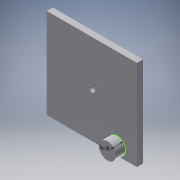
# Autodesk Inventor part: Base
Saved by Autodesk Inventor 2016 SP1 (Build 200210100, 210)
## iProperties
Created: 2016-01-27
Part Number: Base
Material: PVC, non plastifié
Document SubType Name: Modeling
Designer: sd
Density: 1.4 g/cm^3
Appearance: Lisse - Blanc
Author: sd
Autodesk Inventor part; units mm, degrees
ref_plane "YZ Plane" through (0, 0, 0) normal (1, 0, 0) x (0, 1, 0)
ref_plane "XZ Plane" through (0, 0, 0) normal (0, 1, 0) x (-1, 0, 0)
ref_plane "XY Plane" through (0, 0, 0) normal (0, 0, 1) x (1, 0, 0)
sketch "Esquisse1" plane through (0, 0, 0) normal (0, 1, 0) x (-1, 0, 0)
  line L0 (-75, 75) -> (75, 75)
  line L1 (75, 75) -> (75, -75)
  line L2 (75, -75) -> (-75, -75)
  line L3 (-75, -75) -> (-75, 75)
  point P0 (0, 0)
  dimension "d0" = 150
  dimension "d1" = 75
  dimension "d2" = 150
  dimension "d3" = 75
  constraints: 8 end point, 2 parallel, 1 horizontal, 1 perpendicular
  measures "d0" distance of L2.end L0.start
  measures "d1" horizontal distance of point (0, 0) L0.start
  measures "d2" distance of L0.start L0.end
  measures "d3" horizontal distance of point (0, 0) L0.start
extrude "Extrusion1" add sketch "Esquisse1" along normal blind 10
sketch "Esquisse2" plane through (0, 10, 0) normal (0, 1, 0) x (1, 0, 0)
  circle A0 centre (0, 0) radius 5
  dimension "d6" = 10
  constraints: 1 centre point, 1 coincident
  measures "d6" diameter of A0
extrude "Extrusion2" cut sketch "Esquisse2" against normal through all
sketch "Esquisse4" plane through (0, 0, 0) normal (0, -1, 0) x (1, 0, 0)
  circle A0 centre (-65, 65) radius 2
  circle A1 centre (65, 65) radius 2
  circle A2 centre (65, -65) radius 2
  circle A3 centre (-65, -65) radius 2
  line L0 (-75, 75) -> (-75, -75) projected
  line L1 (75, -75) -> (75, 75) projected
  line L2 (75, 75) -> (-75, 75) projected
  line L3 (-75, -75) -> (75, -75) projected
  point P0 (0, 0)
  dimension "d12" = 4
  dimension "d13" = 4
  dimension "d14" = 4
  dimension "d15" = 4
  dimension "d16" = 10
  dimension "d17" = 10
  dimension "d18" = 10
  dimension "d19" = 10
  dimension "d20" = 10
  dimension "d21" = 10
  dimension "d22" = 10
  dimension "d23" = 10
  constraints: 4 centre point
  measures "d12" diameter of A0
  measures "d13" diameter of A1
  measures "d14" diameter of A3
  measures "d15" diameter of A2
  measures "d16" distance from line of L0 A0.centre
  measures "d17" distance from line of L0 A3.centre
  measures "d18" distance from line of L1 A1.centre
  measures "d19" distance from line of L1 A2.centre
  measures "d20" distance from line of A0.centre L2
  measures "d21" distance from line of A1.centre L2
  measures "d22" distance from line of A2.centre L3
  measures "d23" distance from line of A3.centre L3
extrude "Extrusion4" cut sketch "Esquisse4" against normal blind 1 contours A0 | A1 | A2 | A3
equation "\"d1\" = 0.5 * d0"
equation "\"d3\" = 0.5 * d2"
equation "\"d13\" = d12"
equation "\"d14\" = d12"
equation "\"d15\" = d12"
equation "\"d17\" = d16"
equation "\"d18\" = d16"
equation "\"d19\" = d16"
equation "\"d20\" = d16"
equation "\"d21\" = d16"
equation "\"d22\" = d16"
equation "\"d23\" = d16"
equation "\"dd0\" = 16"
equation "\"dd1\" = 28"
